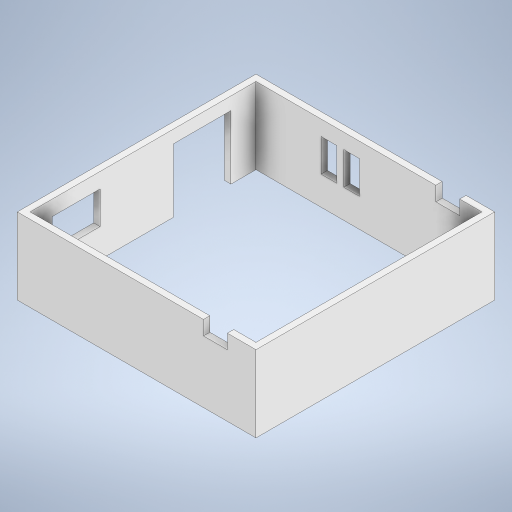
# Autodesk Inventor part: Walls--Exterior--Basement
Saved by Autodesk Inventor 2024 (Build 280153000, 153)
## iProperties
Created: 2023-05-13
Part Number: Walls--Exterior--Basement
Material: Generic
Document SubType Name: Modeling
Designer: Tom
Density: 1 g/cm^3
Appearance: White
Author: Tom
Autodesk Inventor part; units mm, degrees
ref_plane "YZ Plane" through (0, 0, 0) normal (1, 0, 0) x (0, 1, 0)
ref_plane "XZ Plane" through (0, 0, 0) normal (0, 1, 0) x (-1, 0, 0)
ref_plane "XY Plane" through (0, 0, 0) normal (0, 0, 1) x (1, 0, 0)
sketch "Sketch2" plane through (0, 0, 0) normal (0, 1, 0) x (-1, 0, 0)
  line L0 (3810, 3810) -> (-3810, 3810)
  line L1 (-3810, 3810) -> (-3810, -3810)
  line L2 (-3810, -3810) -> (3810, -3810)
  line L3 (3810, -3810) -> (3810, 3810)
  line L4 (3606.8, 3606.8) -> (-3606.8, 3606.8)
  line L5 (-3606.8, 3606.8) -> (-3606.8, -3606.8)
  line L6 (-3606.8, -3606.8) -> (3606.8, -3606.8)
  line L7 (3606.8, -3606.8) -> (3606.8, 3606.8)
  line L8 (3810, 3810) -> (-3810, -3810)
  line L9 (3810, -3810) -> (-3810, 3810)
  point P0 (0, 0)
  point P1 (0, 0)
  point P2 (0, 0)
  dimension "d7" = 7620
  dimension "d8" = 7620
  dimension "d9" = 203.2
  constraints: 20 end point, 4 parallel, 2 coincident, 2 perpendicular, 1 horizontal, 1 midpoint, 3 other
  measures "d7" distance of L2.end L0.start
  measures "d8" distance of L1.end L2.end
  measures "d9" distance between parallel lines of L7 L3
extrude "Extrusion2" add sketch "Sketch2" along normal blind 2438.4 contours L8 L4 L9 L0 | L3 L9 L7 L8 | L9 L5 L8 L1 | L2 L8 L6 L9
sketch "Sketch4" plane through (-3810, 0, 3810) normal (0, 0, 1) x (1, 0, 0)
  line L0 (7416.8, 2438.4) -> (203.2, 2438.4) projected
  line L1 (6705.6, 2438.4) -> (5943.6, 2438.4)
  line L2 (5943.6, 2438.4) -> (5943.6, 1981.2)
  line L3 (5943.6, 1981.2) -> (6705.6, 1981.2)
  line L4 (6705.6, 1981.2) -> (6705.6, 2438.4)
  line L5 (7620, 0) -> (7620, 2438.4) projected
  point P0 (3810, 0)
  point P1 (4622.8, 2438.4)
  dimension "d34" = 914.4
  dimension "d35" = 457.2
  dimension "d36" = 762
  constraints: 8 end point, 2 parallel, 1 horizontal, 1 perpendicular, 1 point on line
  measures "d34" distance between parallel lines of L4 L5
  measures "d35" distance of L1.end L2.end
  measures "d36" distance of L2.end L3.end
extrude "Extrusion4" cut sketch "Sketch4" against normal up to surface (203.2 mm away)
sketch "Sketch5" plane through (3606.8, 0, -3606.8) normal (0, 0, 1) x (1, 0, 0)
  line L0 (-4413.25, 1955.8) -> (-3905.25, 1955.8)
  line L1 (-3905.25, 1955.8) -> (-3905.25, 914.4)
  line L2 (-3905.25, 914.4) -> (-4413.25, 914.4)
  line L3 (-4413.25, 914.4) -> (-4413.25, 1955.8)
  line L4 (-7213.6, 0) -> (0, 0) projected
  point P0 (-3606.8, 0)
  point P1 (0, 2438.4)
  dimension "d40" = 1041.4
  dimension "d42" = 508
  dimension "d43" = 914.4
  dimension "d48" = 3905.25
  constraints: 8 end point, 2 parallel, 1 horizontal, 1 perpendicular
  measures "d40" distance of L0.end L1.end
  measures "d42" distance of L0.start L0.end
  measures "d43" distance between parallel lines of L4 L2
  measures "d48" distance from line of point (0, 2438.4) L1
extrude "Extrusion5" cut sketch "Sketch5" against normal up to surface (203.2 mm away)
sketch "Sketch6" plane through (-3606.8, 0, -3606.8) normal (0, 0, 1) x (1, 0, 0)
  line L0 (0, 2438.4) -> (7213.6, 2438.4) projected
  line L1 (6502.4, 2438.4) -> (5740.4, 2438.4)
  line L2 (5740.4, 2438.4) -> (5740.4, 1981.2)
  line L3 (5740.4, 1981.2) -> (6502.4, 1981.2)
  line L4 (6502.4, 1981.2) -> (6502.4, 2438.4)
  line L5 (7213.6, 0) -> (7213.6, 2438.4) projected
  point P0 (3606.8, 0)
  point P1 (7416.8, 2438.4)
  dimension "d49" = 457.2
  dimension "d50" = 762
  dimension "d52" = 914.4
  constraints: 8 end point, 2 parallel, 1 horizontal, 1 perpendicular, 1 point on line
  measures "d49" distance of L1.end L2.end
  measures "d50" distance of L2.end L3.end
  measures "d52" distance from line of point (7416.8, 2438.4) L4
extrude "Extrusion6" cut sketch "Sketch6" against normal up to surface (203.2 mm away)
sketch "Sketch7" plane through (-3606.8, 0, -3606.8) normal (0, 0, 1) x (1, 0, 0)
  line L0 (2584.45, 1955.8) -> (2076.45, 1955.8)
  line L1 (2076.45, 1955.8) -> (2076.45, 914.4)
  line L2 (2076.45, 914.4) -> (2584.45, 914.4)
  line L3 (2584.45, 914.4) -> (2584.45, 1955.8)
  line L4 (0, 0) -> (0, 2438.4) projected
  line L5 (0, 0) -> (7213.6, 0) projected
  point P0 (3606.8, 0)
  dimension "d55" = 2076.45
  dimension "d57" = 508
  dimension "d58" = 1041.4
  dimension "d59" = 914.4
  constraints: 8 end point, 2 parallel, 1 horizontal, 1 perpendicular
  measures "d55" distance between parallel lines of L4 L1
  measures "d57" distance of L0.start L0.end
  measures "d58" distance of L2.end L0.start
  measures "d59" distance between parallel lines of L5 L2
extrude "Extrusion7" cut sketch "Sketch7" against normal up to surface (203.2 mm away)
sketch "Sketch8" plane through (-3606.8, 0, 3606.8) normal (1, 0, 0) x (0, 0, -1)
  line L0 (0, 0) -> (7213.6, 0) projected
  line L1 (6413.5, 0) -> (4584.7, 0)
  line L2 (4584.7, 0) -> (4584.7, 2032)
  line L3 (4584.7, 2032) -> (6413.5, 2032)
  line L4 (6413.5, 2032) -> (6413.5, 0)
  line L5 (7213.6, 0) -> (7213.6, 2438.4) projected
  point P0 (3606.8, 0)
  point P1 (4584.7, 0)
  dimension "d62" = 800.1
  dimension "d63" = 2032
  dimension "d64" = 1828.8
  constraints: 8 end point, 2 parallel, 1 horizontal, 1 perpendicular, 1 point on line
  measures "d62" distance between parallel lines of L5 L4
  measures "d63" distance of L1.end L2.end
  measures "d64" distance of L2.end L3.end
extrude "Extrusion8" cut sketch "Sketch8" against normal up to surface (203.2 mm away)
sketch "Sketch9" plane through (-3810, 0, 3810) normal (-1, 0, 0) x (0, 0, 1)
  line L0 (-914.4, 1955.8) -> (-2438.4, 1955.8)
  line L1 (-2438.4, 1955.8) -> (-2438.4, 914.4)
  line L2 (-2438.4, 914.4) -> (-914.4, 914.4)
  line L3 (-914.4, 914.4) -> (-914.4, 1955.8)
  line L4 (0, 0) -> (0, 2438.4) projected
  line L5 (-4787.9, 0) -> (0, 0) projected
  point P0 (-3810, 0)
  dimension "d67" = 914.4
  dimension "d68" = 914.4
  dimension "d69" = 1041.4
  dimension "d70" = 1524
  constraints: 8 end point, 2 parallel, 1 horizontal, 1 perpendicular
  measures "d67" distance between parallel lines of L4 L3
  measures "d68" distance between parallel lines of L5 L2
  measures "d69" distance of L0.end L1.end
  measures "d70" distance of L0.start L0.end
extrude "Extrusion9" cut sketch "Sketch9" against normal up to surface (203.2 mm away)
body "Solid2"
